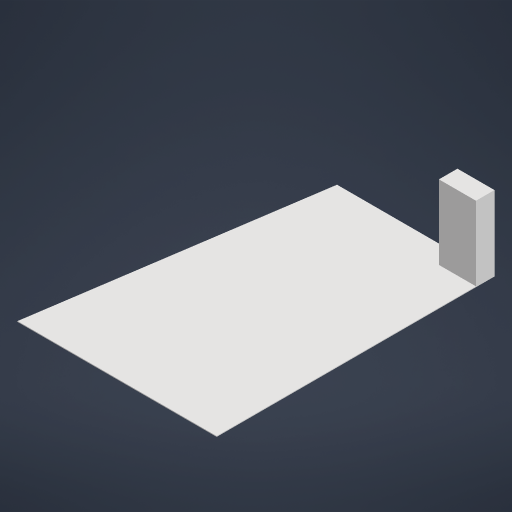
# Autodesk Inventor part: Building
Saved by Autodesk Inventor 2023.1 (Build 271208000, 208)
## iProperties
Created: 2022-11-15
Part Number: Building
Material: Generic
Document SubType Name: Modeling
Designer: aubrey-work
Density: 1 g/cm^3
Appearance: Default
Author: aubrey-work
Autodesk Inventor part; units mm, degrees
ref_plane "YZ Plane" through (0, 0, 0) normal (1, 0, 0) x (0, 1, 0)
ref_plane "XZ Plane" through (0, 0, 0) normal (0, 1, 0) x (-1, 0, 0)
ref_plane "XY Plane" through (0, 0, 0) normal (0, 0, 1) x (1, 0, 0)
sketch "Sketch1" plane through (0, 0, 0) normal (0, 1, 0) x (-1, 0, 0)
  line L0 (0, 0) -> (-1371.6, -9144)
  line L1 (-1371.6, -9144) -> (-6553.2, -9144)
  line L2 (-6553.2, -9144) -> (-6553.2, 0)
  line L3 (-6553.2, 0) -> (-1371.6, 0)
  line L4 (-1371.6, 0) -> (0, 0)
  line L5 (-1371.6, 0) -> (-1371.6, -9144) construction
  line L6 (-6553.2, -9144) -> (-5334, -9144)
  line L7 (-5334, -9144) -> (-5334, -8534.4)
  line L8 (-5334, -8534.4) -> (-6553.2, -8534.4)
  line L9 (-6553.2, -8534.4) -> (-6553.2, -9144)
  dimension "d4" = 1371.6
  dimension "d5" = 9144
  dimension "d6" = 5181.6
  dimension "d7" = 1219.2
  dimension "d8" = 609.6
  constraints: 20 end point, 4 horizontal, 2 parallel, 2 perpendicular, 1 coincident, 1 vertical
  measures "d4" distance of L3.end L0.start
  measures "d5" distance of L3.end L0.end
  measures "d6" distance of L0.end L1.end
  measures "d7" distance of L8.end L7.end
  measures "d8" distance of L7.end L6.end
extrude "Extrusion1" add sketch "Sketch1" against normal blind 25.4
extrude "Extrusion2" add sketch "Sketch1" along normal blind 2438.4 contours L1 L2 L8 L7
equation "\"pillar\" = pillarHeight"
equation "\"pillarHeight\" = 2438.4"
body "Solid1"
